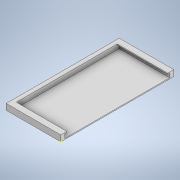
# Autodesk Inventor part: 零件1
Saved by Autodesk Inventor 2022.5 (Build 265521000, 521)
## iProperties
Created: 2024-12-27
Part Number: 零件1
Material: 常规
Document SubType Name: Modeling
Designer: Administrator
Density: 1 g/cm^3
Appearance: 默认
Author: Administrator
Autodesk Inventor part; units mm, degrees
ref_plane "YZ Plane" through (0, 0, 0) normal (1, 0, 0) x (0, 1, 0)
ref_plane "XZ Plane" through (0, 0, 0) normal (0, 1, 0) x (-1, 0, 0)
ref_plane "XY Plane" through (0, 0, 0) normal (0, 0, 1) x (1, 0, 0)
sketch "草图1" plane through (0, 0, 0) normal (0, 1, 0) x (-1, 0, 0)
  line L0 (0, 0) -> (27, 0)
  line L1 (27, 0) -> (27, -56)
  line L2 (27, -56) -> (0, -56)
  line L3 (0, -56) -> (0, 0)
  dimension "d0" = 27
  dimension "d1" = 56
  constraints: 8 end point, 2 parallel, 1 horizontal, 1 perpendicular
  measures "d0" distance of L1.end L2.end
  measures "d1" distance of L0.end L1.end
extrude "拉伸1" add sketch "草图1" along normal blind 3
sketch "草图2" plane through (0, 0, 0) normal (1, 0, 0) x (0, 0, -1)
  line L0 (56, 3) -> (0, 3) projected
  line L1 (28, 3) -> (28, -4.4631)
  line L2 (19.0299, 3) -> (19.0299, 2.5)
  line L3 (28, 2.5) -> (2, 2.5)
  line L4 (2, 2.5) -> (2, 0.5)
  line L5 (2, 0.5) -> (28, 0.5)
  line L6 (28, 0.5) -> (28, 2.5)
  point P0 (0, 0)
  dimension "d4" = 0.5
  dimension "d5" = 26
  dimension "d6" = 2
  constraints: 12 end point, 2 parallel, 2 point on line, 2 vertical, 1 horizontal, 1 midpoint, 1 perpendicular
  measures "d4" distance of L2.start L2.end
  measures "d5" distance of L5.end L4.end
  measures "d6" distance of L4.end L3.end
extrude "拉伸2" cut sketch "草图2" against normal blind 25 contours L1 L5 L4 L3
mirror "镜像1" about plane through (0, 2.5, -28) normal (0, 0, 1) of "拉伸2"
sketch "草图3" plane through (0, 0, 0) normal (1, 0, 0) x (0, 0, -1)
  point P0 (0, 0)
sketch "草图4" plane through (0, 0, 0) normal (1, 0, 0) x (0, 0, -1)
  line L0 (56, 3) -> (0, 3) projected
  line L1 (28, 3) -> (28, -1.1507)
  line L2 (28, 3) -> (3, 3)
  line L3 (3, 3) -> (3, 2.5)
  line L4 (54, 2.5) -> (2, 2.5) projected
  line L5 (0, 0) -> (56, 0) projected
  line L6 (56, 0) -> (56, 3) projected
  line L7 (0, 3) -> (56, 3) projected
  line L8 (0, 0) -> (0, 3) projected
  line L9 (2, 2.5) -> (54, 2.5) projected
  line L10 (54, 2.5) -> (54, 0.5) projected
  line L11 (54, 0.5) -> (2, 0.5) projected
  line L12 (2, 0.5) -> (2, 2.5) projected
  point P0 (28, 2.5)
  dimension "d9" = 25
  constraints: 6 end point, 2 point on line, 2 vertical, 1 midpoint
  measures "d9" distance of L1.start L2.end
extrude "拉伸3" cut sketch "草图4" against normal blind 25 contours L1 L4 L3 L0
mirror "镜像2" about plane through (0, 3, -28) normal (0, 0, 1) of "拉伸3"
